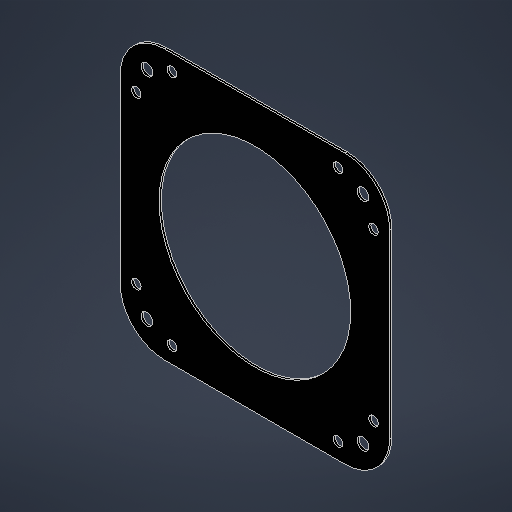
# Autodesk Inventor part: stator_mount_02_left_p
Saved by Autodesk Inventor 2026.1 (Build 301233000, 233)
## iProperties
Created: 2026-04-12
Part Number: stator_mount_02_left_p
Material: PC/ABS Plastic
Document SubType Name: Modeling
Designer: aaron
Density: 1.1 g/cm^3
Appearance: Smooth - White
Author: aaron
Autodesk Inventor part; units mm, degrees
ref_plane "YZ Plane" through (0, 0, 0) normal (1, 0, 0) x (0, 1, 0)
ref_plane "XZ Plane" through (0, 0, 0) normal (0, 1, 0) x (-1, 0, 0)
ref_plane "XY Plane" through (0, 0, 0) normal (0, 0, 1) x (1, 0, 0)
sketch "Sketch1" plane through (0, 0, 0) normal (0, 0, 1) x (1, 0, 0)
  circle A0 centre (0, 0) radius 29
  circle A1 centre (0, 0) radius 60.5
  line L0 (-40.5, 60.5) -> (40.5, 60.5)
  line L1 (60.5, 40.5) -> (60.5, -40.5)
  line L2 (40.5, -60.5) -> (-40.5, -60.5)
  line L3 (-60.5, -40.5) -> (-60.5, 40.5)
  arc A2 (-40.5, 60.5) -> (-60.5, 40.5) centre (-40.5, 40.5) ccw
  arc A3 (60.5, 40.5) -> (40.5, 60.5) centre (40.5, 40.5) ccw
  arc A4 (40.5, -60.5) -> (60.5, -40.5) centre (40.5, -40.5) ccw
  arc A5 (-60.5, -40.5) -> (-40.5, -60.5) centre (-40.5, -40.5) ccw
  dimension "d0" = 58
  dimension "d1" = 121
  dimension "d2" = 20
  constraints: 12 tangent, 8 end point, 8 point on circle, 6 centre point, 3 equal radius, 2 coincident, 2 parallel, 1 horizontal, 1 perpendicular
  measures "d0" diameter of A0
  measures "d1" diameter of A1
  measures "d2" radius of A2
extrude "Extrusion1" add sketch "Sketch1" along normal blind 1
sketch "Sketch2" plane through (0, 0, 1) normal (0, 0, 1) x (1, 0, 0)
  circle A0 centre (-48.4865, -48.5066) radius 2.65 projected
  circle A1 centre (-37.2683, -53.25) radius 2.15 projected
  circle A2 centre (-53.2329, -37.2897) radius 2.15 projected
  circle A3 centre (-53.2431, 37.2752) radius 2.15 projected
  circle A4 centre (-48.4997, 48.4934) radius 2.65 projected
  circle A5 centre (-37.2829, 53.2398) radius 2.15 projected
  circle A6 centre (37.2821, 53.25) radius 2.15 projected
  circle A7 centre (48.5003, 48.5066) radius 2.65 projected
  circle A8 centre (53.2467, 37.2897) radius 2.15 projected
  circle A9 centre (53.2569, -37.2752) radius 2.15 projected
  circle A10 centre (48.5135, -48.4934) radius 2.65 projected
  circle A11 centre (37.2966, -53.2398) radius 2.15 projected
  point P0 (0, 0)
extrude "Extrusion2" cut sketch "Sketch2" against normal through all
sketch "Sketch3" plane through (0, 0, 0) normal (0, 0, -1) x (-1, 0, 0)
  circle A0 centre (-0.0069, 0) radius 43 projected
  point P0 (0, 0)
extrude "Extrusion3" cut sketch "Sketch3" against normal through all
body "Solid1"
